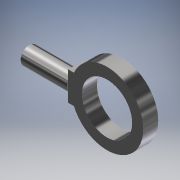
# Autodesk Inventor part: M6 Eye Bolt
Saved by Autodesk Inventor 2019.4 (Build 234330000, 330)
## iProperties
Created: 2020-01-24
Part Number: M6 Eye Bolt
Material: Stainless Steel
Document SubType Name: Modeling
Designer: Mark
Mass: 14.7283 g
Surface Area: 15.5275 cm^2
Volume: 1.84103 cm^3
Density: 8 g/cm^3
Appearance: Semi-Polished
Author: Mark
Autodesk Inventor part; units mm, degrees
ref_plane "YZ Plane" through (0, 0, 0) normal (1, 0, 0) x (0, 1, 0)
ref_plane "XZ Plane" through (0, 0, 0) normal (0, 1, 0) x (-1, 0, 0)
ref_plane "XY Plane" through (0, 0, 0) normal (0, 0, 1) x (1, 0, 0)
sketch "Sketch1" plane through (0, 0, 0) normal (0, 0, 1) x (1, 0, 0)
  circle A0 centre (0, 0) radius 8.69
  arc A1 (-11.5, -4.899) -> (-11.5, 4.899) centre (0, 0) ccw
  line L0 (-13.5, 5) -> (-11.5, 5)
  line L1 (-11.5, 5) -> (-11.5, -5)
  line L2 (-11.5, -5) -> (-13.5, -5)
  line L3 (-13.5, -5) -> (-13.5, 5)
  line L4 (-13.5, 5) -> (-11.5, -5) construction
  line L5 (-11.5, 5) -> (-13.5, -5) construction
  dimension "d0" = 17.38
  dimension "d1" = 25
  dimension "d4" = 2
  dimension "d5" = 10
  constraints: 12 end point, 2 centre point, 2 coincident, 2 parallel, 2 point on circle, 2 point on line, 1 horizontal, 1 perpendicular
  measures "d0" diameter of A0
  measures "d1" diameter of A1
  measures "d4" distance of L1.end L2.end
  measures "d5" distance of L0.end L1.end
extrude "Extrusion1" add sketch "Sketch1" along normal blind 5.2
sketch "Sketch2" plane through (-13.5, -5, 0) normal (-1, 0, 0) x (0, 0, 1)
  circle A0 centre (2.6, 5) radius 3
  line L0 (5.2, 10) -> (5.2, 0) projected
  line L1 (0, 0) -> (5.2, 0) projected
  point P0 (0, 5)
  dimension "d6" = 6
  dimension "d7" = 2.6
  dimension "d8" = 5
  constraints: 1 centre point
  measures "d6" diameter of A0
  measures "d7" distance from line of L0 A0.centre
  measures "d8" distance from line of L1 A0.centre
extrude "Extrusion2" add sketch "Sketch2" along normal blind 16
body "Solid1"
